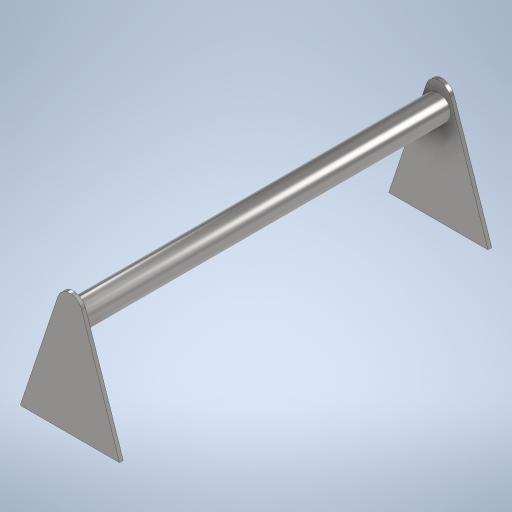
# Autodesk Inventor part: stand
Saved by Autodesk Inventor 2023 (Build 270158030, 158C)
## iProperties
Created: 2024-01-19
Part Number: stand
Material: Generic
Document SubType Name: Modeling
Designer: HP
Density: 1 g/cm^3
Appearance: Default
Author: HP
Autodesk Inventor part; units mm, degrees
ref_plane "YZ Plane" through (0, 0, 0) normal (1, 0, 0) x (0, 1, 0)
ref_plane "XZ Plane" through (0, 0, 0) normal (0, 1, 0) x (-1, 0, 0)
ref_plane "XY Plane" through (0, 0, 0) normal (0, 0, 1) x (1, 0, 0)
sketch "Sketch1" plane through (0, 0, 0) normal (0, 0, 1) x (1, 0, 0)
  point P0 (0, 0)
sketch "Sketch2" plane through (0, 0, 0) normal (0, 0, 1) x (1, 0, 0)
  line L0 (0, 0) -> (80, 0)
  line L1 (80, 0) -> (40, 120)
  line L2 (40, 120) -> (0, 0)
  dimension "d0" = 80
  dimension "d1" = 120
  dimension "d2" = 40
  constraints: 6 end point, 1 horizontal
  measures "d0" distance of L0.start L0.end
  measures "d1" distance from line of L0 L1.end
  measures "d2" horizontal distance of L0.start L1.end
extrude "Extrusion1" add sketch "Sketch2" against normal blind 3
sketch "Sketch3" plane through (0, 0, -3) normal (0, 0, -1) x (-1, 0, 0)
  circle A0 centre (-40, 80) radius 10
  line L0 (-80, 0) -> (0, 0) projected
  point P0 (-40, 120)
  point P1 (-40, 0)
  dimension "d5" = 20
  dimension "d6" = 0
  dimension "d7" = 80
  constraints: 1 centre point, 1 midpoint
  measures "d5" diameter of A0
  measures "d6" horizontal distance of point (-40, 120) A0.centre
  measures "d7" distance of point (-40, 0) A0.centre
fillet "Fillet1" radius 10 1 edges at (40, 120, -1.5)
extrude "Extrusion2" add sketch "Sketch3" along normal blind 147
mirror "Mirror1" about plane through (40, 80, -150) normal (0, 0, -1) of "Extrusion2", "Extrusion1"
fillet "Fillet2" radius 10 1 edges at (40, 120, -298.5)
body "Solid1"
